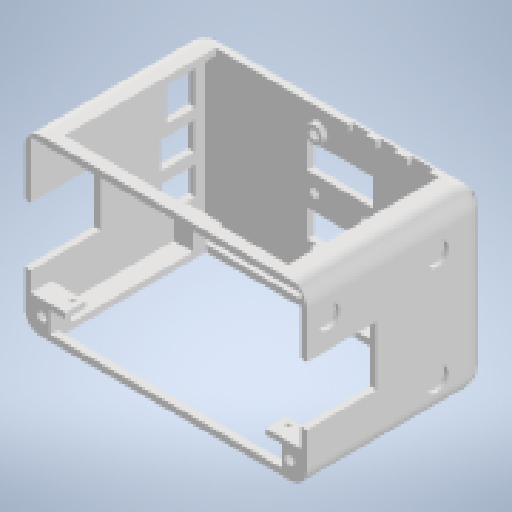
# Autodesk Inventor part: лицо
Saved by Autodesk Inventor 2024.2 (Build 282272000, 272)
## iProperties
Created: 2025-10-19
Part Number: лицо
Material: Типовые
Document SubType Name: Modeling
Designer: katya_notebook
Density: 1 g/cm^3
Appearance: По умолчанию
Author: katya_notebook
Autodesk Inventor part; units mm, degrees
ref_plane "YZ Plane" through (0, 0, 0) normal (1, 0, 0) x (0, 1, 0)
ref_plane "XZ Plane" through (0, 0, 0) normal (0, 1, 0) x (-1, 0, 0)
ref_plane "XY Plane" through (0, 0, 0) normal (0, 0, 1) x (1, 0, 0)
sketch "Эскиз1" plane through (0, 0, 0) normal (0, 0, 1) x (1, 0, 0)
  line L0 (-65, -40) -> (65, -40)
  line L1 (65, -40) -> (65, 40)
  line L2 (65, 40) -> (-65, 40)
  line L3 (-65, 40) -> (-65, -40)
  line L4 (-65, -40) -> (65, 40) construction
  line L5 (65, -40) -> (-65, 40) construction
  point P0 (0, 0)
  dimension "d0" = 80
  dimension "d1" = 130
  constraints: 12 end point, 2 midpoint, 2 parallel, 1 horizontal, 1 perpendicular
  measures "d0" distance of L0.end L1.end
  measures "d1" distance of L1.end L2.end
extrude "Выдавливание1" add sketch "Эскиз1" along normal blind 3
sketch "Эскиз2" plane through (0, 0, 3) normal (0, 0, 1) x (1, 0, 0)
  line L0 (-62, -37) -> (62, -37)
  line L1 (62, -37) -> (62, 37)
  line L2 (62, 37) -> (-62, 37)
  line L3 (-62, 37) -> (-62, -37)
  line L4 (-62, -37) -> (62, 37) construction
  line L5 (62, -37) -> (-62, 37) construction
  line L6 (-65, -40) -> (65, -40)
  line L7 (65, -40) -> (65, 40)
  line L8 (65, 40) -> (-65, 40)
  line L9 (-65, 40) -> (-65, -40)
  line L10 (-65, -40) -> (65, 40) construction
  line L11 (65, -40) -> (-65, 40) construction
  point P0 (0, 0)
  dimension "d8" = 3
  dimension "d9" = 3
  constraints: 24 end point, 4 midpoint, 4 parallel, 2 horizontal, 2 perpendicular
  measures "d8" distance between parallel lines of L7 L1
  measures "d9" distance between parallel lines of L2 L8
extrude "Выдавливание2" add sketch "Эскиз2" along normal blind 80
fillet "Сопряжение1" radius 8 8 edges at (-65, 40, 41.5) (-65, -40, 41.5) (65, -40, 41.5) (65, 40, 41.5) (-65, 0, 0) (0, -40, 0) (65, 0, 0) (0, 40, 0)
sketch "Эскиз3" plane through (-57, -40, 8) normal (0, -1, 0) x (1, 0, 0)
  line L0 (110, 71.5) -> (4, 71.5) projected
  line L1 (4, 71.5) -> (4, 3.5) projected
  line L2 (4, 71.5) -> (110, 71.5)
  line L3 (4, 3.36) -> (4, 71.5)
  line L4 (57, 71.5) -> (57, 3.5)
  line L5 (4, 37.43) -> (110.34, 37.43)
  line L6 (110.34, 3.36) -> (4, 3.36)
  line L7 (4, 3.36) -> (4, 71.5)
  line L8 (4, 71.5) -> (110.34, 71.5)
  line L9 (110.34, 71.5) -> (110.34, 3.36)
  line L10 (110.34, 3.36) -> (4, 71.5) construction
  line L11 (4, 3.36) -> (110.34, 71.5) construction
  point P0 (57, -8)
  point P1 (57.17, 37.43)
  point P2 (4, 3.5)
  point P3 (4, 3.36)
  dimension "d16" = 106.34
  dimension "d17" = 68.14
  constraints: 20 end point, 5 midpoint, 2 horizontal, 2 parallel, 1 perpendicular
  measures "d16" distance of L6.start L6.end
  measures "d17" distance of L8.end L6.start
extrude "Выдавливание3" cut sketch "Эскиз3" against normal blind 12
sketch "Эскиз4" plane through (0, 0, 0) normal (0, 0, -1) x (-1, 0, 0)
  circle A0 centre (11.8725, 0) radius 2 projected
  circle A1 centre (-11.8725, 0) radius 2 projected
  line L0 (15, -19.9954) -> (-15, -19.9954) construction
  line L1 (15, -7.4954) -> (15, -19.9954) construction
  line L2 (-15, -7.4954) -> (15, -7.4954) construction
  line L3 (-15, -19.9954) -> (-15, -7.4954) construction
  circle A2 centre (11.8725, 0) radius 2
  circle A3 centre (-11.8725, 0) radius 2
  line L4 (-15, -7.4954) -> (15, -7.4954)
  line L5 (15, -7.4954) -> (15, -19.9954)
  line L6 (15, -19.9954) -> (-15, -19.9954)
  line L7 (-15, -19.9954) -> (-15, -7.4954)
  line L8 (-15, -7.4954) -> (15, -19.9954) construction
  line L9 (15, -7.4954) -> (-15, -19.9954) construction
  line L10 (20.0944, 0) -> (-19.4677, 0)
  line L11 (15, 19.9954) -> (-15, 19.9954) construction
  line L12 (15, 7.4954) -> (15, 19.9954) construction
  line L13 (-15, 7.4954) -> (15, 7.4954) construction
  line L14 (-15, 19.9954) -> (-15, 7.4954) construction
  line L15 (-15, 19.9954) -> (15, 19.9954)
  line L16 (15, 19.9954) -> (15, 7.4954)
  line L17 (15, 7.4954) -> (-15, 7.4954)
  line L18 (-15, 7.4954) -> (-15, 19.9954)
  line L19 (-15, 19.9954) -> (15, 7.4954) construction
  line L20 (15, 19.9954) -> (-15, 7.4954) construction
  point P0 (0, 0)
  point P1 (0, -13.7454)
  point P2 (0, 13.7454)
  constraints: 34 end point, 4 midpoint, 4 parallel, 4 symmetric about line, 3 horizontal, 2 centre point, 2 coincident, 2 concentric, 2 perpendicular
extrude "Выдавливание4" cut sketch "Эскиз4" against normal blind 10
sketch "Эскиз5" plane through (-62, -37, 3) normal (0, 1, 0) x (1, 0, 0)
  circle A0 centre (111.7, -73.45) radius 2.75 projected
  circle A1 centre (12.5, -73.45) radius 2.75 projected
  circle A2 centre (111.7, -11.55) radius 2.75 projected
  circle A3 centre (12.5, -11.55) radius 2.75 projected
  line L0 (115.2, -76.5) -> (115.2, -8.5) projected
  line L1 (9, -8.5) -> (9, -76.5) projected
  line L2 (115.34, -76.5) -> (9, -76.5) projected
  line L3 (115.34, -8.36) -> (115.34, -76.5) projected
  line L4 (115.34, -76.5) -> (125.34, -76.5)
  line L5 (125.34, -76.5) -> (125.34, -70.5)
  line L6 (125.34, -70.5) -> (115.34, -70.5)
  line L7 (115.34, -70.5) -> (115.34, -76.5)
  line L8 (9, -8.36) -> (115.34, -8.36) projected
  line L9 (115.34, -8.36) -> (125.34, -8.36)
  line L10 (125.34, -8.36) -> (125.34, -14.36)
  line L11 (125.34, -14.36) -> (115.34, -14.36)
  line L12 (115.34, -14.36) -> (115.34, -8.36)
  line L13 (9, -76.5) -> (-1, -76.5)
  line L14 (-1, -76.5) -> (-1, -70.5)
  line L15 (-1, -70.5) -> (9, -70.5)
  line L16 (9, -70.5) -> (9, -76.5)
  line L17 (9, -76.5) -> (9, -8.36) projected
  line L18 (9, -8.36) -> (-1, -8.36)
  line L19 (-1, -8.36) -> (-1, -14.36)
  line L20 (-1, -14.36) -> (9, -14.36)
  line L21 (9, -14.36) -> (9, -8.36)
  point P0 (62, 3)
  point P1 (9, -14.36)
  point P2 (9, -70.5)
  dimension "d20" = 6
  dimension "d21" = 10
  dimension "d22" = 10
  dimension "d23" = 6
  dimension "d24" = 6
  dimension "d25" = 10
  dimension "d26" = 10
  dimension "d27" = 6
  constraints: 32 end point, 8 parallel, 4 horizontal, 4 perpendicular
  measures "d20" distance of L4.end L5.end
  measures "d21" distance of L5.end L6.end
  measures "d22" distance of L10.end L11.end
  measures "d23" distance of L9.end L10.end
  measures "d24" distance of L13.end L14.end
  measures "d25" distance of L1.end L13.end
  measures "d26" distance of L19.end L20.end
  measures "d27" distance of L18.end L19.end
ref_plane "РабПлоскость1" through (-52.25, -27.4, 73.7) normal (0, 1, 0) x (0, 0, 1)
extrude "Выдавливание5" add sketch "Эскиз5" along normal up to surface (9.6 mm away) contours L1 L20 L19 L18 L17 | L1 L13 L14 L15 | L9 L10 L11 L3 | L6 L5 L4 L3
ref_plane "РабПлоскость2" through (0.1, -27.4, 2.5765) normal (0, 1, 0) x (1, 0, 0)
sketch "Эскиз6" plane through (0.1, -27.4, 2.5765) normal (0, 1, 0) x (1, 0, 0)
  circle A0 centre (49.6, -73.8735) radius 1 projected
  circle A1 centre (-49.6, -73.8735) radius 1 projected
  circle A2 centre (-49.6, -11.9735) radius 1 projected
  circle A3 centre (49.6, -11.9735) radius 1 projected
  line L0 (61.9, -76.9235) -> (53.24, -76.9235) projected
  line L1 (61.9, -70.9235) -> (61.9, -76.9235) projected
  line L2 (61.9, -76.9235) -> (45.9, -76.9235)
  line L3 (45.9, -76.9235) -> (45.9, -70.9235)
  line L4 (45.9, -70.9235) -> (61.9, -70.9235)
  line L5 (61.9, -70.9235) -> (61.9, -76.9235)
  circle A4 centre (49.6, -73.8735) radius 1
  line L6 (61.9, -14.7835) -> (53.24, -14.7835) projected
  line L7 (61.9, -8.7835) -> (61.9, -14.7835) projected
  line L8 (-53.1, -76.9235) -> (-62.1, -76.9235) projected
  line L9 (-62.1, -76.9235) -> (-62.1, -70.9235) projected
  line L10 (-62.1, -14.7835) -> (-62.1, -8.7835) projected
  line L11 (-53.1, -14.7835) -> (-62.1, -14.7835) projected
  line L12 (61.9, -14.7835) -> (45.9, -14.7835)
  line L13 (45.9, -14.7835) -> (45.9, -8.7835)
  line L14 (45.9, -8.7835) -> (61.9, -8.7835)
  line L15 (61.9, -8.7835) -> (61.9, -14.7835)
  circle A5 centre (49.6, -11.9735) radius 1
  circle A6 centre (-49.6, -73.8735) radius 1
  circle A7 centre (-49.6, -11.9735) radius 1
  line L16 (-62.1, -76.9235) -> (-46.1, -76.9235)
  line L17 (-46.1, -76.9235) -> (-46.1, -70.9235)
  line L18 (-46.1, -70.9235) -> (-62.1, -70.9235)
  line L19 (-62.1, -70.9235) -> (-62.1, -76.9235)
  line L20 (-62.1, -14.7835) -> (-46.1, -14.7835)
  line L21 (-46.1, -14.7835) -> (-46.1, -8.7835)
  line L22 (-46.1, -8.7835) -> (-62.1, -8.7835)
  line L23 (-62.1, -8.7835) -> (-62.1, -14.7835)
  point P0 (-0.1, 2.5765)
  point P1 (61.9, -8.7835)
  point P2 (61.9, -70.9235)
  point P3 (53.24, -76.9235)
  point P4 (-62.1, -70.9235)
  dimension "d30" = 16
  dimension "d31" = 16
  dimension "d32" = 6
  dimension "d33" = 16
  dimension "d34" = 16
  constraints: 32 end point, 8 parallel, 4 centre point, 4 coincident, 4 concentric, 4 horizontal, 4 perpendicular
  measures "d30" distance of L3.end L4.end
  measures "d31" distance of L13.end L14.end
  measures "d32" distance of L16.end L17.end
  measures "d33" distance of L17.end L18.end
  measures "d34" distance of L10.start L20.end
extrude "Выдавливание6" add sketch "Эскиз6" along normal blind 2.5
sketch "Эскиз7" plane through (65, -32, 83) normal (1, 0, 0) x (0, 0, -1)
  line L0 (6.631, 19.5) -> (-99.237, 19.5) projected
  line L1 (6.631, 39.5) -> (-99.237, 39.5) projected
  line L2 (-8, 16) -> (0, 16) projected
  line L3 (0, 43) -> (-8, 43) projected
  line L4 (-8, 16) -> (32, 16)
  line L5 (32, 16) -> (32, 43)
  line L6 (32, 43) -> (-8, 43)
  line L7 (-8, 16) -> (-8, 43)
  point P0 (83, 32)
  point P1 (0, 16)
  dimension "d39" = 40
  constraints: 8 end point, 2 perpendicular, 1 collinear, 1 horizontal
  measures "d39" distance of L2.start L4.end
extrude "Выдавливание7" cut sketch "Эскиз7" against normal blind 162
sketch "Эскиз8" plane through (0, 0, 3) normal (0, 0, 1) x (1, 0, 0)
  circle A0 centre (-9.5, -23.5) radius 1.35 projected
  circle A1 centre (48.5, -23.5) radius 1.3 projected
  circle A2 centre (-9.5, 25.5) radius 1.35 projected
  circle A3 centre (48.5, 25.5) radius 1.35 projected
  circle A4 centre (-9.5, -23.5) radius 2.1
  circle A5 centre (48.5, 25.5) radius 2.1
  circle A6 centre (-9.5, 25.5) radius 2.1
  circle A7 centre (48.5, -23.5) radius 2.1
  point P0 (0, 0)
  dimension "d42" = 4.2
  dimension "d43" = 4.2
  dimension "d44" = 4.2
  dimension "d45" = 4.2
  constraints: 4 centre point, 4 coincident
  measures "d42" diameter of A4
  measures "d43" diameter of A5
  measures "d44" diameter of A6
  measures "d45" diameter of A7
extrude "Выдавливание8" cut sketch "Эскиз8" against normal blind 10 contours A0 | A1 | A2 | A3 | A4 | A5 | A6 | A7
sketch "Эскиз9" plane through (-65, -32, 8) normal (-1, 0, 0) x (0, 0, 1)
  line L0 (14.55, 7.55) -> (14.55, 20.45) projected
  line L1 (15.13, 25.65) -> (15.13, 38.15) projected
  line L2 (12.45, 58.55) -> (12.45, 43.05) projected
  line L3 (12.45, 43.05) -> (-0.55, 43.05)
  line L4 (-0.55, 43.05) -> (-0.55, 58.55)
  line L5 (-0.55, 58.55) -> (12.45, 58.55)
  line L6 (12.45, 58.55) -> (12.45, 43.05)
  line L7 (15.13, 38.15) -> (-0.12, 38.15)
  line L8 (-0.12, 38.15) -> (-0.12, 25.65)
  line L9 (-0.12, 25.65) -> (15.13, 25.65)
  line L10 (15.13, 25.65) -> (15.13, 38.15)
  line L11 (14.55, 20.45) -> (-0.55, 20.45)
  line L12 (-0.55, 20.45) -> (-0.55, 7.55)
  line L13 (-0.55, 7.55) -> (14.55, 7.55)
  line L14 (14.55, 7.55) -> (14.55, 20.45)
  point P0 (1.8, 49.7575)
  point P1 (2.38, 45.4575)
  point P2 (1.95, 27.8075)
  constraints: 24 end point, 6 parallel, 3 horizontal, 3 perpendicular, 3 other
extrude "Выдавливание9" cut sketch "Эскиз9" against normal blind 10
sketch "Эскиз10" plane through (-57, 40, 83) normal (0, 1, 0) x (1, 0, 0)
  line L0 (94.63, 72.89) -> (100.97, 72.89) projected
  line L1 (80.4, 73.15) -> (86, 73.15) projected
  line L2 (67, 73.15) -> (72.6, 73.15) projected
  line L3 (100.97, 72.89) -> (92.9118, 72.89)
  line L4 (92.9118, 72.89) -> (92.9118, 77.3203)
  line L5 (92.9118, 77.3203) -> (100.9456, 77.3203)
  line L6 (86, 73.15) -> (79.0834, 73.15)
  line L7 (79.0834, 73.15) -> (79.0834, 76.9507)
  line L8 (79.0834, 76.9507) -> (85.7857, 76.9507)
  line L9 (72.6, 73.15) -> (66.0508, 73.15)
  line L10 (66.0508, 73.15) -> (66.0508, 76.9507)
  line L11 (66.0508, 76.9507) -> (72.6, 76.9507)
  line L12 (100.97, 72.89) -> (102.9243, 72.89)
  line L13 (102.9243, 72.89) -> (102.9243, 77.3203)
  line L14 (102.9243, 77.3203) -> (100.97, 77.3203)
  line L15 (86, 73.15) -> (87.1846, 73.15)
  line L16 (87.1846, 73.15) -> (87.1846, 76.9507)
  line L17 (114, 75) -> (0, 75) projected
  line L18 (87.1846, 76.9507) -> (85.7857, 76.9507)
  line L19 (72.6, 73.15) -> (73.8677, 73.15)
  line L20 (73.8677, 73.15) -> (73.8677, 76.9507)
  line L21 (73.8677, 76.9507) -> (72.6, 76.9507)
  line L22 (100.97, 77.3203) -> (100.9456, 77.3203)
  point P0 (57, 83)
  point P1 (86.45, 72.4202)
  point P2 (94.63, 70.39)
  point P3 (80.4, 70.65)
  point P4 (67, 70.65)
  point P5 (101.1231, 74.3133)
  constraints: 38 end point, 7 perpendicular, 6 horizontal, 3 parallel, 3 point on line, 1 other
extrude "Выдавливание10" cut sketch "Эскиз10" against normal blind 10
sketch "Эскиз11" plane through (-57, 40, 83) normal (0, 1, 0) x (1, 0, 0)
  circle A0 centre (106.7, 6.55) radius 1 projected
  circle A1 centre (106.7, 68.45) radius 1 projected
  circle A2 centre (7.5, 6.55) radius 1 projected
  circle A3 centre (7.5, 68.45) radius 1 projected
  line L0 (0, 75) -> (114, 75) projected
  line L1 (107.7, 75) -> (4.9791, 75)
  line L2 (4.9791, 75) -> (4.9791, 5.55)
  line L3 (4.9791, 5.55) -> (107.7, 5.55)
  line L4 (107.7, 5.55) -> (107.7, 75)
  point P0 (57, 83)
  point P1 (4.9791, 75)
  constraints: 8 end point, 2 parallel, 1 horizontal, 1 perpendicular, 1 point on line
extrude "Выдавливание11" cut sketch "Эскиз11" against normal blind 10 contours A0 | L4 L3 A0 | A1 | A2 | A0 L3 L2 L0 L4 | A3
sketch "Эскиз12" plane through (65, -32, 8) normal (1, 0, 0) x (0, 0, -1)
  circle A0 centre (-65, 6) radius 5
  circle A1 centre (-65, 56) radius 5
  circle A2 centre (-15, 6) radius 5
  circle A3 centre (-15, 56) radius 5
  line L0 (-43, 16) -> (-75, 16) projected
  line L1 (-75, 0) -> (-75, 16) projected
  point P0 (8, 32)
  point P1 (-59, 16)
  dimension "d52" = 10
  dimension "d53" = 10
  dimension "d54" = 10
  dimension "d55" = 50
  dimension "d56" = 0
  dimension "d57" = 0
  dimension "d58" = 50
  dimension "d59" = 50
  dimension "d60" = 0
  constraints: 4 centre point, 3 equal radius, 1 midpoint
  measures "d52" diameter of A0
  measures "d53" vertical distance of point (-59, 16) A0.centre
  measures "d54" distance from line of L1 A0.centre
  measures "d55" distance of A2.centre A0.centre
  measures "d56" vertical distance of A2.centre A0.centre
  measures "d57" horizontal distance of A2.centre A3.centre
  measures "d58" distance of A3.centre A2.centre
  measures "d59" distance of A1.centre A3.centre
  measures "d60" vertical distance of A3.centre A1.centre
extrude "Выдавливание12" cut sketch "Эскиз12" against normal blind 2
sketch "Эскиз13" plane through (-65, -32, 8) normal (-1, 0, 0) x (0, 0, 1)
  circle A0 centre (65, 6) radius 5 projected
  circle A1 centre (65, 56) radius 5 projected
  circle A2 centre (25, 56) radius 5
  circle A3 centre (25, 6) radius 5
  point P0 (-8, 32)
  dimension "d63" = 40
  dimension "d64" = 50
  dimension "d65" = 0
  constraints: 2 centre point, 2 equal radius
  measures "d63" distance of A2.centre A1.centre
  measures "d64" distance of A2.centre A3.centre
  measures "d65" horizontal distance of A2.centre A3.centre
extrude "Выдавливание13" cut sketch "Эскиз13" against normal blind 2
sketch "Эскиз14" plane through (0, 0, 3) normal (0, 0, 1) x (1, 0, 0)
  circle A0 centre (48.5, 25.5) radius 2.1 projected
  circle A1 centre (-9.5, 25.5) radius 2.1 projected
  circle A2 centre (-9.5, -23.5) radius 2.1 projected
  circle A3 centre (48.5, -23.5) radius 2.1 projected
  circle A4 centre (48.5, 25.5) radius 2.1 projected
  circle A5 centre (48.5, 25.5) radius 4
  circle A6 centre (-9.5, 25.5) radius 4
  circle A7 centre (-9.5, -23.5) radius 3.505
  circle A8 centre (48.5, -23.5) radius 4
  point P0 (0, 0)
  point P1 (46, -24.9)
  dimension "d68" = 8
  dimension "d69" = 7.01
  constraints: 4 centre point, 4 coincident, 2 equal radius
  measures "d68" diameter of A5
  measures "d69" diameter of A7
extrude "Выдавливание14" add sketch "Эскиз14" along normal blind 2.5
sketch "Эскиз15" plane through (0, 0, 0) normal (0, 0, -1) x (-1, 0, 0)
  circle A0 centre (-48.5, 25.5) radius 2.1 projected
  circle A1 centre (-48.5, -23.5) radius 2.1 projected
  circle A2 centre (9.5, -23.5) radius 2.1 projected
  circle A3 centre (9.5, 25.5) radius 2.1 projected
  point P0 (0, 0)
extrude "Выдавливание15" add sketch "Эскиз15" against normal blind 0.5
sketch "Эскиз16" plane through (53.34, -37, 79.5) normal (0, 0, 1) x (1, 0, 0)
  line L0 (8.66, 12.1) -> (8.66, 0) projected
  line L1 (-7.34, 12.1) -> (8.66, 12.1) projected
  line L2 (-7.34, 9.6) -> (-7.34, 12.1) projected
  line L3 (-7.34, 9.6) -> (0, 9.6) projected
  line L4 (0, 0) -> (0, 9.6) projected
  line L5 (8.66, 0) -> (0, 0) projected
  line L6 (-115.34, 0) -> (-115.34, 12.1) projected
  line L7 (-106.34, 0) -> (-115.34, 0) projected
  line L8 (-106.34, 0) -> (-106.34, 9.6) projected
  line L9 (-106.34, 9.6) -> (-99.34, 9.6) projected
  line L10 (-99.34, 9.6) -> (-99.34, 12.1) projected
  line L11 (-115.34, 12.1) -> (-99.34, 12.1) projected
  point P0 (-53.34, 37)
extrude "Выдавливание16" add sketch "Эскиз16" along normal up to surface (3.5 mm away)
sketch "Эскиз17" plane through (0, 0, 83) normal (0, 0, 1) x (1, 0, 0)
  circle A0 centre (57, -32) radius 2.1
  line L0 (65, -32) -> (65, -16) projected
  circle A1 centre (-57, -32) radius 2.1
  line L1 (-57, -40) -> (57, -40) projected
  line L2 (-53, -27.4) -> (-53, -37) projected
  point P0 (0, 0)
  dimension "d76" = 8
  dimension "d77" = 8
  dimension "d78" = 4.2
  dimension "d79" = 8
  dimension "d80" = 4
  dimension "d81" = 4.2
  constraints: 2 centre point
  measures "d76" distance of L1.end A0.centre
  measures "d77" distance from line of L0 A0.centre
  measures "d78" diameter of A0
  measures "d79" distance from line of L1 A1.centre
  measures "d80" distance from line of L2 A1.centre
  measures "d81" diameter of A1
extrude "Выдавливание17" cut sketch "Эскиз17" against normal blind 5
sketch "Эскиз18" plane through (63, -26, 73) normal (1, 0, 0) x (0, 0, -1)
  circle A0 centre (0, 0) radius 5 projected
  point P0 (73, 26)
extrude "Выдавливание18" add sketch "Эскиз18" along normal blind 2
sketch "Эскиз19" plane through (-63, -26, 73) normal (-1, 0, 0) x (0, 0, 1)
  circle A0 centre (0, 0) radius 5 projected
  point P0 (-73, 26)
extrude "Выдавливание19" add sketch "Эскиз19" along normal blind 2
